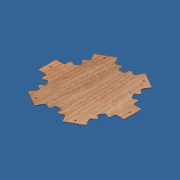
# Autodesk Inventor part: BaseTop
Saved by Autodesk Inventor 2014 SP2 (Build 180246200, 246)
## iProperties
Created: 2015-02-08
Part Number: BaseTop
Material: Holz (Birke)
Document SubType Name: Modeling
Designer: 4ndreas
Density: 0.55 g/cm^3
Appearance: Birke - natur - poliert
Author: 4ndreas
Autodesk Inventor part; units mm, degrees
ref_plane "YZ Plane" through (0, 0, 0) normal (1, 0, 0) x (0, 1, 0)
ref_plane "XZ Plane" through (0, 0, 0) normal (0, 1, 0) x (-1, 0, 0)
ref_plane "XY Plane" through (0, 0, 0) normal (0, 0, 1) x (1, 0, 0)
sketch "Skizze1" plane through (0, 0, 0) normal (0, 0, 1) x (1, 0, 0)
  arc A0 (67.0189, -1.4199) -> (65.1888, 5.4103) centre (62.6888, 1.0801) ccw projected
  line L0 (65.1888, 5.4103) -> (49.6003, 14.4103) projected
  line L1 (49.6003, 14.4103) -> (37.2798, 17.75) projected
  line L2 (37.2798, 17.75) -> (17.2798, 17.75) projected
  line L3 (17.2798, 17.75) -> (4.9593, 14.4103) projected
  line L4 (4.9593, 14.4103) -> (-10.6292, 5.4103) projected
  arc A1 (-10.6292, 5.4103) -> (-12.4593, -1.4199) centre (-8.1292, 1.0801) ccw projected
  line L5 (-12.4593, -1.4199) -> (-4.4593, -15.2763) projected
  arc A2 (-4.4593, -15.2763) -> (2.3708, -17.1064) centre (-0.1292, -12.7763) ccw projected
  line L6 (2.3708, -17.1064) -> (9.7798, -12.8288) projected
  arc A3 (17.2798, -17.159) -> (9.7798, -12.8288) centre (12.2798, -17.159) ccw projected
  line L7 (17.2798, -17.159) -> (17.2798, -23.4987) projected
  arc A4 (17.2798, -23.4987) -> (22.2798, -28.4987) centre (22.2798, -23.4987) ccw projected
  line L8 (22.2798, -28.4987) -> (32.2798, -28.4987) projected
  arc A5 (32.2798, -28.4987) -> (37.2798, -23.4987) centre (32.2798, -23.4987) ccw projected
  line L9 (37.2798, -23.4987) -> (37.2798, -17.159) projected
  arc A6 (44.7798, -12.8288) -> (37.2798, -17.159) centre (42.2798, -17.159) ccw projected
  line L10 (44.7798, -12.8288) -> (52.1888, -17.1064) projected
  arc A7 (52.1888, -17.1064) -> (59.0189, -15.2763) centre (54.6888, -12.7763) ccw projected
  line L11 (59.0189, -15.2763) -> (67.0189, -1.4199) projected
  circle A8 centre (27.2798, 7.75) radius 5.5 projected
  circle A9 centre (27.2798, -18.4987) radius 5.5 projected
  circle A10 centre (54.5596, 0) radius 5.5 projected
  circle A11 centre (0, 0) radius 5.5 projected
  arc A12 (-59.2247, -28.4199) -> (-66.0548, -26.5897) centre (-63.5548, -30.9199) ccw projected
  line L12 (-66.0548, -26.5897) -> (-81.6432, -35.5897) projected
  line L13 (-81.6432, -35.5897) -> (-90.6958, -44.5897) projected
  line L14 (-90.6958, -44.5897) -> (-100.6958, -61.9103) projected
  line L15 (-100.6958, -61.9103) -> (-103.9638, -74.25) projected
  line L16 (-103.9638, -74.25) -> (-103.9638, -92.25) projected
  arc A13 (-103.9638, -92.25) -> (-98.9638, -97.25) centre (-98.9638, -92.25) ccw projected
  line L17 (-98.9638, -97.25) -> (-82.9638, -97.25) projected
  arc A14 (-82.9638, -97.25) -> (-77.9638, -92.25) centre (-82.9638, -92.25) ccw projected
  line L18 (-77.9638, -92.25) -> (-77.9638, -83.6949) projected
  arc A15 (-70.4638, -79.3647) -> (-77.9638, -83.6949) centre (-72.9638, -83.6949) ccw projected
  line L19 (-70.4638, -79.3647) -> (-64.9734, -82.5346) projected
  arc A16 (-64.9734, -82.5346) -> (-58.1432, -80.7045) centre (-62.4734, -78.2045) ccw projected
  line L20 (-58.1432, -80.7045) -> (-53.1432, -72.0442) projected
  arc A17 (-53.1432, -72.0442) -> (-54.9734, -65.2141) centre (-57.4734, -69.5442) ccw projected
  line L21 (-54.9734, -65.2141) -> (-60.4638, -62.0442) projected
  arc A18 (-60.4638, -53.384) -> (-60.4638, -62.0442) centre (-57.9638, -57.7141) ccw projected
  line L22 (-60.4638, -53.384) -> (-53.0548, -49.1064) projected
  arc A19 (-53.0548, -49.1064) -> (-51.2247, -42.2763) centre (-55.5548, -44.7763) ccw projected
  line L23 (-51.2247, -42.2763) -> (-59.2247, -28.4199) projected
  circle A20 centre (-87.0356, -58.25) radius 5.5 projected
  circle A21 centre (-64.3035, -71.3744) radius 5.5 projected
  circle A22 centre (-66.684, -38.5) radius 5.5 projected
  circle A23 centre (-93.9638, -85.75) radius 5.5 projected
  arc A24 (-98.9638, -151.25) -> (-103.9638, -156.25) centre (-98.9638, -156.25) ccw projected
  line L24 (-103.9638, -156.25) -> (-103.9638, -174.25) projected
  line L25 (-103.9638, -174.25) -> (-100.6958, -186.5897) projected
  line L26 (-100.6958, -186.5897) -> (-90.6958, -203.9103) projected
  line L27 (-90.6958, -203.9103) -> (-81.6432, -212.9103) projected
  line L28 (-81.6432, -212.9103) -> (-66.0548, -221.9103) projected
  arc A25 (-66.0548, -221.9103) -> (-59.2247, -220.0801) centre (-63.5548, -217.5801) ccw projected
  line L29 (-59.2247, -220.0801) -> (-51.2247, -206.2237) projected
  arc A26 (-51.2247, -206.2237) -> (-53.0548, -199.3936) centre (-55.5548, -203.7237) ccw projected
  line L30 (-53.0548, -199.3936) -> (-60.4638, -195.116) projected
  arc A27 (-60.4638, -186.4558) -> (-60.4638, -195.116) centre (-57.9638, -190.7859) ccw projected
  line L31 (-60.4638, -186.4558) -> (-54.9734, -183.2859) projected
  arc A28 (-54.9734, -183.2859) -> (-53.1432, -176.4558) centre (-57.4734, -178.9558) ccw projected
  line L32 (-53.1432, -176.4558) -> (-58.1432, -167.7955) projected
  arc A29 (-58.1432, -167.7955) -> (-64.9734, -165.9654) centre (-62.4734, -170.2955) ccw projected
  line L33 (-64.9734, -165.9654) -> (-70.4638, -169.1353) projected
  arc A30 (-77.9638, -164.8051) -> (-70.4638, -169.1353) centre (-72.9638, -164.8051) ccw projected
  line L34 (-77.9638, -164.8051) -> (-77.9638, -156.25) projected
  arc A31 (-77.9638, -156.25) -> (-82.9638, -151.25) centre (-82.9638, -156.25) ccw projected
  line L35 (-82.9638, -151.25) -> (-98.9638, -151.25) projected
  circle A32 centre (-87.0356, -190.25) radius 5.5 projected
  circle A33 centre (-64.3035, -177.1256) radius 5.5 projected
  circle A34 centre (-93.9638, -162.75) radius 5.5 projected
  circle A35 centre (-66.684, -210) radius 5.5 projected
  arc A36 (-12.4593, -247.0801) -> (-10.6292, -253.9103) centre (-8.1292, -249.5801) ccw projected
  line L36 (-10.6292, -253.9103) -> (4.9593, -262.9103) projected
  line L37 (4.9593, -262.9103) -> (17.2798, -266.25) projected
  line L38 (17.2798, -266.25) -> (37.2798, -266.25) projected
  line L39 (37.2798, -266.25) -> (49.6003, -262.9103) projected
  line L40 (49.6003, -262.9103) -> (65.1888, -253.9103) projected
  arc A37 (65.1888, -253.9103) -> (67.0189, -247.0801) centre (62.6888, -249.5801) ccw projected
  line L41 (67.0189, -247.0801) -> (59.0189, -233.2237) projected
  arc A38 (59.0189, -233.2237) -> (52.1888, -231.3936) centre (54.6888, -235.7237) ccw projected
  line L42 (52.1888, -231.3936) -> (44.7798, -235.6712) projected
  arc A39 (37.2798, -231.341) -> (44.7798, -235.6712) centre (42.2798, -231.341) ccw projected
  line L43 (37.2798, -231.341) -> (37.2798, -225.0013) projected
  arc A40 (37.2798, -225.0013) -> (32.2798, -220.0013) centre (32.2798, -225.0013) ccw projected
  line L44 (32.2798, -220.0013) -> (22.2798, -220.0013) projected
  arc A41 (22.2798, -220.0013) -> (17.2798, -225.0013) centre (22.2798, -225.0013) ccw projected
  line L45 (17.2798, -225.0013) -> (17.2798, -231.341) projected
  arc A42 (9.7798, -235.6712) -> (17.2798, -231.341) centre (12.2798, -231.341) ccw projected
  line L46 (9.7798, -235.6712) -> (2.3708, -231.3936) projected
  arc A43 (2.3708, -231.3936) -> (-4.4593, -233.2237) centre (-0.1292, -235.7237) ccw projected
  line L47 (-4.4593, -233.2237) -> (-12.4593, -247.0801) projected
  circle A44 centre (27.2798, -256.25) radius 5.5 projected
  circle A45 centre (27.2798, -230.0013) radius 5.5 projected
  circle A46 centre (0, -248.5) radius 5.5 projected
  circle A47 centre (54.5596, -248.5) radius 5.5 projected
  arc A48 (113.7843, -220.0801) -> (120.6144, -221.9103) centre (118.1144, -217.5801) ccw projected
  line L48 (120.6144, -221.9103) -> (136.2028, -212.9103) projected
  line L49 (136.2028, -212.9103) -> (145.2554, -203.9103) projected
  line L50 (145.2554, -203.9103) -> (155.2554, -186.5897) projected
  line L51 (155.2554, -186.5897) -> (158.5234, -174.25) projected
  line L52 (158.5234, -174.25) -> (158.5234, -156.25) projected
  arc A49 (158.5234, -156.25) -> (153.5234, -151.25) centre (153.5234, -156.25) ccw projected
  line L53 (153.5234, -151.25) -> (137.5234, -151.25) projected
  arc A50 (137.5234, -151.25) -> (132.5234, -156.25) centre (137.5234, -156.25) ccw projected
  line L54 (132.5234, -156.25) -> (132.5234, -164.8051) projected
  arc A51 (125.0234, -169.1353) -> (132.5234, -164.8051) centre (127.5234, -164.8051) ccw projected
  line L55 (125.0234, -169.1353) -> (119.533, -165.9654) projected
  arc A52 (119.533, -165.9654) -> (112.7028, -167.7955) centre (117.033, -170.2955) ccw projected
  line L56 (112.7028, -167.7955) -> (107.7028, -176.4558) projected
  arc A53 (107.7028, -176.4558) -> (109.533, -183.2859) centre (112.033, -178.9558) ccw projected
  line L57 (109.533, -183.2859) -> (115.0234, -186.4558) projected
  arc A54 (115.0234, -195.116) -> (115.0234, -186.4558) centre (112.5234, -190.7859) ccw projected
  line L58 (115.0234, -195.116) -> (107.6144, -199.3936) projected
  arc A55 (107.6144, -199.3936) -> (105.7843, -206.2237) centre (110.1144, -203.7237) ccw projected
  line L59 (105.7843, -206.2237) -> (113.7843, -220.0801) projected
  circle A56 centre (141.5952, -190.25) radius 5.5 projected
  circle A57 centre (118.8631, -177.1256) radius 5.5 projected
  circle A58 centre (121.2436, -210) radius 5.5 projected
  circle A59 centre (148.5234, -162.75) radius 5.5 projected
  arc A60 (153.5234, -97.25) -> (158.5234, -92.25) centre (153.5234, -92.25) ccw projected
  line L60 (158.5234, -92.25) -> (158.5234, -74.25) projected
  line L61 (158.5234, -74.25) -> (155.2554, -61.9103) projected
  line L62 (155.2554, -61.9103) -> (145.2554, -44.5897) projected
  line L63 (145.2554, -44.5897) -> (136.2028, -35.5897) projected
  line L64 (136.2028, -35.5897) -> (120.6144, -26.5897) projected
  arc A61 (120.6144, -26.5897) -> (113.7843, -28.4199) centre (118.1144, -30.9199) ccw projected
  line L65 (113.7843, -28.4199) -> (105.7843, -42.2763) projected
  arc A62 (105.7843, -42.2763) -> (107.6144, -49.1064) centre (110.1144, -44.7763) ccw projected
  line L66 (107.6144, -49.1064) -> (115.0234, -53.384) projected
  arc A63 (115.0234, -62.0442) -> (115.0234, -53.384) centre (112.5234, -57.7141) ccw projected
  line L67 (115.0234, -62.0442) -> (109.533, -65.2141) projected
  arc A64 (109.533, -65.2141) -> (107.7028, -72.0442) centre (112.033, -69.5442) ccw projected
  line L68 (107.7028, -72.0442) -> (112.7028, -80.7045) projected
  arc A65 (112.7028, -80.7045) -> (119.533, -82.5346) centre (117.033, -78.2045) ccw projected
  line L69 (119.533, -82.5346) -> (125.0234, -79.3647) projected
  arc A66 (132.5234, -83.6949) -> (125.0234, -79.3647) centre (127.5234, -83.6949) ccw projected
  line L70 (132.5234, -83.6949) -> (132.5234, -92.25) projected
  arc A67 (132.5234, -92.25) -> (137.5234, -97.25) centre (137.5234, -92.25) ccw projected
  line L71 (137.5234, -97.25) -> (153.5234, -97.25) projected
  circle A68 centre (141.5952, -58.25) radius 5.5 projected
  circle A69 centre (118.8631, -71.3744) radius 5.5 projected
  circle A70 centre (148.5234, -85.75) radius 5.5 projected
  circle A71 centre (121.2436, -38.5) radius 5.5 projected
  line L72 (-37.254, -137.2494) -> (-38.7651, -138.1242) projected
  arc A72 (-38.7651, -138.1242) -> (-40.345, -144.0482) centre (-13.7095, -147.9791) ccw projected
  line L73 (-40.345, -144.0482) -> (-23.5645, -173.0347) projected
  arc A73 (-23.5645, -173.0347) -> (-17.6405, -174.6146) centre (-13.7095, -147.9791) ccw projected
  line L74 (-17.6405, -174.6146) -> (-16.1294, -173.7398) projected
  arc A74 (-16.1294, -173.7398) -> (-37.254, -137.2494) centre (27.2798, -124.25) ccw projected
  circle A75 centre (27.2798, -124.25) radius 80 projected
  arc A76 (-5.9641, -110.8301) -> (-4.134, -117.6603) centre (-1.634, -113.3301) ccw projected
  line L75 (-0.9641, -102.1699) -> (-5.9641, -110.8301) projected
  arc A77 (5.866, -100.3397) -> (-0.9641, -102.1699) centre (3.366, -104.6699) ccw projected
  line L76 (18.8564, -107.8397) -> (5.866, -100.3397) projected
  line L77 (35.7032, -107.8397) -> (18.8564, -107.8397) projected
  line L78 (35.7032, -107.8397) -> (48.6936, -100.3397) projected
  arc A78 (55.5237, -102.1699) -> (48.6936, -100.3397) centre (51.1936, -104.6699) ccw projected
  line L79 (60.5237, -110.8301) -> (55.5237, -102.1699) projected
  arc A79 (58.6936, -117.6603) -> (60.5237, -110.8301) centre (56.1936, -113.3301) ccw projected
  line L80 (45.7032, -125.1603) -> (58.6936, -117.6603) projected
  line L81 (37.2798, -139.75) -> (45.7032, -125.1603) projected
  line L82 (37.2798, -139.75) -> (37.2798, -154.75) projected
  arc A80 (32.2798, -159.75) -> (37.2798, -154.75) centre (32.2798, -154.75) ccw projected
  line L83 (22.2798, -159.75) -> (32.2798, -159.75) projected
  arc A81 (17.2798, -154.75) -> (22.2798, -159.75) centre (22.2798, -154.75) ccw projected
  line L84 (17.2798, -139.75) -> (17.2798, -154.75) projected
  line L85 (8.8564, -125.1603) -> (17.2798, -139.75) projected
  line L86 (8.8564, -125.1603) -> (-4.134, -117.6603) projected
  circle A82 centre (27.2798, -149.75) radius 5.5 projected
  circle A83 centre (49.3634, -111.5) radius 5.5 projected
  circle A84 centre (5.1962, -111.5) radius 5.5 projected
  circle A85 centre (27.2798, -124.25) radius 11.5 projected
  arc A86 (-38.7651, -138.1242) -> (-40.345, -144.0482) centre (-13.7095, -147.9791) ccw projected
  line L87 (-9.7786, -121.3436) -> (-38.7651, -138.1242) projected
  arc A87 (-3.8546, -122.9235) -> (-9.7786, -121.3436) centre (-13.7095, -147.9791) ccw projected
  line L88 (12.926, -151.91) -> (-3.8546, -122.9235) projected
  arc A88 (11.346, -157.8341) -> (12.926, -151.91) centre (-13.7095, -147.9791) ccw projected
  line L89 (-17.6405, -174.6146) -> (11.346, -157.8341) projected
  arc A89 (-23.5645, -173.0347) -> (-17.6405, -174.6146) centre (-13.7095, -147.9791) ccw projected
  line L90 (-40.345, -144.0482) -> (-23.5645, -173.0347) projected
  arc A90 (-15.9365, -144.1322) -> (-11.4825, -151.826) centre (-13.7095, -147.9791) ccw projected
  arc A91 (-11.4825, -151.826) -> (-15.9365, -144.1322) centre (-13.7095, -147.9791) ccw projected
  line L91 (137.5234, -150.65) -> (153.5234, -150.65)
  arc A92 (159.1234, -156.25) -> (153.5234, -150.65) centre (153.5234, -156.25) ccw
  line L92 (159.1234, -156.25) -> (159.1234, -174.3281)
  line L93 (159.1234, -174.3281) -> (155.815, -186.8206)
  line L94 (155.815, -186.8206) -> (145.7351, -204.2794)
  line L95 (145.7351, -204.2794) -> (136.5705, -213.3908)
  line L96 (136.5705, -213.3908) -> (120.9144, -222.4299)
  arc A93 (113.2646, -220.3801) -> (120.9144, -222.4299) centre (118.1144, -217.5801) ccw
  line L97 (113.2646, -220.3801) -> (105.2646, -206.5237)
  arc A94 (107.3144, -198.874) -> (105.2646, -206.5237) centre (110.1144, -203.7237) ccw
  line L98 (107.3144, -198.874) -> (114.7234, -194.5964)
  arc A95 (114.7234, -194.5964) -> (114.7234, -186.9754) centre (112.5234, -190.7859) ccw
  line L99 (114.7234, -186.9754) -> (109.233, -183.8055)
  arc A96 (107.1832, -176.1558) -> (109.233, -183.8055) centre (112.033, -178.9558) ccw
  line L100 (107.1832, -176.1558) -> (112.1832, -167.4955)
  arc A97 (119.833, -165.4458) -> (112.1832, -167.4955) centre (117.033, -170.2955) ccw
  line L101 (119.833, -165.4458) -> (125.3234, -168.6156)
  arc A98 (125.3234, -168.6156) -> (131.9234, -164.8051) centre (127.5234, -164.8051) ccw
  line L102 (131.9234, -164.8051) -> (131.9234, -156.25)
  arc A99 (137.5234, -150.65) -> (131.9234, -156.25) centre (137.5234, -156.25) ccw
  line L103 (131.9234, -92.25) -> (131.9234, -83.6949)
  arc A100 (131.9234, -83.6949) -> (125.3234, -79.8844) centre (127.5234, -83.6949) ccw
  line L104 (125.3234, -79.8844) -> (119.833, -83.0542)
  arc A101 (112.1832, -81.0045) -> (119.833, -83.0542) centre (117.033, -78.2045) ccw
  line L105 (112.1832, -81.0045) -> (107.1832, -72.3442)
  arc A102 (109.233, -64.6945) -> (107.1832, -72.3442) centre (112.033, -69.5442) ccw
  line L106 (109.233, -64.6945) -> (114.7234, -61.5246)
  arc A103 (114.7234, -61.5246) -> (114.7234, -53.9036) centre (112.5234, -57.7141) ccw
  line L107 (114.7234, -53.9036) -> (107.3144, -49.626)
  arc A104 (105.2646, -41.9763) -> (107.3144, -49.626) centre (110.1144, -44.7763) ccw
  line L108 (105.2646, -41.9763) -> (113.2646, -28.1199)
  arc A105 (120.9144, -26.0701) -> (113.2646, -28.1199) centre (118.1144, -30.9199) ccw
  line L109 (120.9144, -26.0701) -> (136.5705, -35.1092)
  line L110 (136.5705, -35.1092) -> (145.7351, -44.2206)
  line L111 (145.7351, -44.2206) -> (155.815, -61.6794)
  line L112 (155.815, -61.6794) -> (159.1234, -74.1719)
  line L113 (159.1234, -74.1719) -> (159.1234, -92.25)
  arc A106 (153.5234, -97.85) -> (159.1234, -92.25) centre (153.5234, -92.25) ccw
  line L114 (153.5234, -97.85) -> (137.5234, -97.85)
  arc A107 (131.9234, -92.25) -> (137.5234, -97.85) centre (137.5234, -92.25) ccw
  line L115 (16.6798, -23.4987) -> (16.6798, -17.159)
  arc A108 (16.6798, -17.159) -> (10.0798, -13.3485) centre (12.2798, -17.159) ccw
  line L116 (10.0798, -13.3485) -> (2.6708, -17.626)
  arc A109 (-4.9789, -15.5763) -> (2.6708, -17.626) centre (-0.1292, -12.7763) ccw
  line L117 (-4.9789, -15.5763) -> (-12.9789, -1.7199)
  arc A110 (-10.9292, 5.9299) -> (-12.9789, -1.7199) centre (-8.1292, 1.0801) ccw
  line L118 (-10.9292, 5.9299) -> (4.7269, 14.9689)
  line L119 (4.7269, 14.9689) -> (17.1999, 18.35)
  line L120 (17.1999, 18.35) -> (37.3597, 18.35)
  line L121 (37.3597, 18.35) -> (49.8327, 14.9689)
  line L122 (49.8327, 14.9689) -> (65.4888, 5.9299)
  arc A111 (67.5385, -1.7199) -> (65.4888, 5.9299) centre (62.6888, 1.0801) ccw
  line L123 (67.5385, -1.7199) -> (59.5385, -15.5763)
  arc A112 (51.8888, -17.626) -> (59.5385, -15.5763) centre (54.6888, -12.7763) ccw
  line L124 (51.8888, -17.626) -> (44.4798, -13.3485)
  arc A113 (44.4798, -13.3485) -> (37.8798, -17.159) centre (42.2798, -17.159) ccw
  line L125 (37.8798, -17.159) -> (37.8798, -23.4987)
  arc A114 (32.2798, -29.0987) -> (37.8798, -23.4987) centre (32.2798, -23.4987) ccw
  line L126 (32.2798, -29.0987) -> (22.2798, -29.0987)
  arc A115 (16.6798, -23.4987) -> (22.2798, -29.0987) centre (22.2798, -23.4987) ccw
  arc A116 (-52.7548, -49.626) -> (-50.705, -41.9763) centre (-55.5548, -44.7763) ccw
  line L127 (-52.7548, -49.626) -> (-60.1638, -53.9036)
  arc A117 (-60.1638, -53.9036) -> (-60.1638, -61.5246) centre (-57.9638, -57.7141) ccw
  line L128 (-60.1638, -61.5246) -> (-54.6734, -64.6945)
  arc A118 (-52.6236, -72.3442) -> (-54.6734, -64.6945) centre (-57.4734, -69.5442) ccw
  line L129 (-52.6236, -72.3442) -> (-57.6236, -81.0045)
  arc A119 (-65.2734, -83.0542) -> (-57.6236, -81.0045) centre (-62.4734, -78.2045) ccw
  line L130 (-65.2734, -83.0542) -> (-70.7638, -79.8844)
  arc A120 (-70.7638, -79.8844) -> (-77.3638, -83.6949) centre (-72.9638, -83.6949) ccw
  line L131 (-77.3638, -83.6949) -> (-77.3638, -92.25)
  arc A121 (-82.9638, -97.85) -> (-77.3638, -92.25) centre (-82.9638, -92.25) ccw
  line L132 (-82.9638, -97.85) -> (-98.9638, -97.85)
  arc A122 (-104.5638, -92.25) -> (-98.9638, -97.85) centre (-98.9638, -92.25) ccw
  line L133 (-104.5638, -92.25) -> (-104.5638, -74.1719)
  line L134 (-104.5638, -74.1719) -> (-101.2554, -61.6794)
  line L135 (-101.2554, -61.6794) -> (-91.1755, -44.2206)
  line L136 (-91.1755, -44.2206) -> (-82.0109, -35.1092)
  line L137 (-82.0109, -35.1092) -> (-66.3548, -26.0701)
  arc A123 (-58.705, -28.1199) -> (-66.3548, -26.0701) centre (-63.5548, -30.9199) ccw
  line L138 (-58.705, -28.1199) -> (-50.705, -41.9763)
  arc A124 (59.5385, -232.9237) -> (51.8888, -230.874) centre (54.6888, -235.7237) ccw
  line L139 (59.5385, -232.9237) -> (67.5385, -246.7801)
  arc A125 (65.4888, -254.4299) -> (67.5385, -246.7801) centre (62.6888, -249.5801) ccw
  line L140 (65.4888, -254.4299) -> (49.8327, -263.4689)
  line L141 (49.8327, -263.4689) -> (37.3597, -266.85)
  line L142 (37.3597, -266.85) -> (17.1999, -266.85)
  line L143 (17.1999, -266.85) -> (4.7269, -263.4689)
  line L144 (4.7269, -263.4689) -> (-10.9292, -254.4299)
  arc A126 (-12.9789, -246.7801) -> (-10.9292, -254.4299) centre (-8.1292, -249.5801) ccw
  line L145 (-12.9789, -246.7801) -> (-4.9789, -232.9237)
  arc A127 (2.6708, -230.874) -> (-4.9789, -232.9237) centre (-0.1292, -235.7237) ccw
  line L146 (2.6708, -230.874) -> (10.0798, -235.1515)
  arc A128 (10.0798, -235.1515) -> (16.6798, -231.341) centre (12.2798, -231.341) ccw
  line L147 (16.6798, -231.341) -> (16.6798, -225.0013)
  arc A129 (22.2798, -219.4013) -> (16.6798, -225.0013) centre (22.2798, -225.0013) ccw
  line L148 (22.2798, -219.4013) -> (32.2798, -219.4013)
  arc A130 (37.8798, -225.0013) -> (32.2798, -219.4013) centre (32.2798, -225.0013) ccw
  line L149 (37.8798, -225.0013) -> (37.8798, -231.341)
  arc A131 (37.8798, -231.341) -> (44.4798, -235.1515) centre (42.2798, -231.341) ccw
  line L150 (44.4798, -235.1515) -> (51.8888, -230.874)
  line L151 (-66.3548, -222.4299) -> (-82.0109, -213.3908)
  line L152 (-82.0109, -213.3908) -> (-91.1755, -204.2794)
  line L153 (-91.1755, -204.2794) -> (-101.2554, -186.8206)
  line L154 (-101.2554, -186.8206) -> (-104.5638, -174.3281)
  line L155 (-104.5638, -174.3281) -> (-104.5638, -156.25)
  arc A132 (-98.9638, -150.65) -> (-104.5638, -156.25) centre (-98.9638, -156.25) ccw
  line L156 (-98.9638, -150.65) -> (-82.9638, -150.65)
  arc A133 (-77.3638, -156.25) -> (-82.9638, -150.65) centre (-82.9638, -156.25) ccw
  line L157 (-77.3638, -156.25) -> (-77.3638, -164.8051)
  arc A134 (-77.3638, -164.8051) -> (-70.7638, -168.6156) centre (-72.9638, -164.8051) ccw
  line L158 (-70.7638, -168.6156) -> (-65.2734, -165.4458)
  arc A135 (-57.6236, -167.4955) -> (-65.2734, -165.4458) centre (-62.4734, -170.2955) ccw
  line L159 (-57.6236, -167.4955) -> (-52.6236, -176.1558)
  arc A136 (-54.6734, -183.8055) -> (-52.6236, -176.1558) centre (-57.4734, -178.9558) ccw
  line L160 (-54.6734, -183.8055) -> (-60.1638, -186.9754)
  arc A137 (-60.1638, -186.9754) -> (-60.1638, -194.5964) centre (-57.9638, -190.7859) ccw
  line L161 (-60.1638, -194.5964) -> (-52.7548, -198.874)
  arc A138 (-50.705, -206.5237) -> (-52.7548, -198.874) centre (-55.5548, -203.7237) ccw
  line L162 (-50.705, -206.5237) -> (-58.705, -220.3801)
  arc A139 (-66.3548, -222.4299) -> (-58.705, -220.3801) centre (-63.5548, -217.5801) ccw
  line L163 (158.5234, -153.7281) -> (158.5234, -94.7719)
  line L164 (118.4304, -25.3288) -> (67.3728, 4.1493)
  line L165 (-12.8132, 4.1493) -> (-63.8708, -25.3288)
  line L166 (-103.9638, -153.7281) -> (-103.9638, -94.7719)
  line L167 (-12.8132, -252.6493) -> (-63.8708, -223.1712)
  line L168 (118.4304, -223.1712) -> (67.3728, -252.6493)
  point P0 (0, 0)
  dimension "d0" = 0.6
  dimension "d1" = 0.6
  dimension "d2" = 0.6
  dimension "d3" = 0.6
  dimension "d4" = 0.6
  dimension "d5" = 0.6
  constraints: 156 end point, 108 point on circle, 48 centre point, 7 collinear, 2 parallel, 114 other
  measures "d0" distance between parallel lines of L53 L91
  measures "d1" distance between parallel lines of L41 L139
  measures "d2" distance between parallel lines of L162 L29
  measures "d3" distance between parallel lines of L132 L17
  measures "d4" distance between parallel lines of L117 L5
  measures "d5" distance between parallel lines of L114 L71
extrude "Extrusion1" add sketch "Skizze1" against normal blind 3 contours A75 | A99 L102 A98 L101 A97 L100 A96 L99 A95 L98 A94 L97 A93 L168 A125 L139 A124 L150 A131 L149 A130 L148 A129 L147 A128 L146 A127 L145 A126 L167 A139 L162 A138 L161 A137 L160 A136 L159 A135 L158 A134 L157 A133 L156 A132 L166 A122 L132 A121 L131 A120 L130 A119 L129 A118 L128 A117 L127 A116 L138 A123 L165 A110 L117 A109 L116 A108 L115 A115 L126 A114 L125 A113 L124 A112 L123 A111 L164 A105 L108 A104 L107 A103 L106 A102 L105 A101 L104 A100 L103 A107 L114 A106 L163 A92 L91
fillet "Rundung1" radius 2 12 edges at (158.5234, -153.7281, -1.5) (158.5234, -94.7719, -1.5) (118.4304, -25.3288, -1.5) (67.3728, 4.1493, -1.5) (-12.8132, 4.1493, -1.5) (-63.8708, -25.3288, -1.5) (-103.9638, -94.7719, -1.5) (-103.9638, -153.7281, -1.5) (-63.8708, -223.1712, -1.5) (-12.8132, -252.6493, -1.5) (67.3728, -252.6493, -1.5) (118.4304, -223.1712, -1.5)
sketch "Skizze2" plane through (0, 0, 0) normal (0, 0, 1) x (1, 0, 0)
  arc A0 (-38.7651, -138.1242) -> (-40.345, -144.0482) centre (-13.7095, -147.9791) ccw
  line L0 (-38.7651, -138.1242) -> (-37.254, -137.2494)
  arc A1 (-16.1294, -173.7398) -> (-37.254, -137.2494) centre (27.2798, -124.25) ccw
  line L1 (-16.1294, -173.7398) -> (-17.6405, -174.6146)
  arc A2 (-23.5645, -173.0347) -> (-17.6405, -174.6146) centre (-13.7095, -147.9791) ccw
  line L2 (-23.5645, -173.0347) -> (-40.345, -144.0482)
  circle A3 centre (27.2798, -124.25) radius 80
  circle A4 centre (27.1946, -51.335) radius 3.3
  circle A5 centre (90.3834, -87.7187) radius 3.3
  circle A6 centre (90.4686, -160.6337) radius 3.3
  circle A7 centre (27.365, -197.165) radius 3.3
  circle A8 centre (-35.8238, -160.7813) radius 3.3
  circle A9 centre (-35.909, -87.8663) radius 3.3
  arc A10 (50.9479, -139.702) -> (49.0131, -139.363) centre (49.4912, -142.3246) ccw
  line L3 (49.0131, -139.363) -> (40.732, -140.7)
  arc A11 (19.7134, -104.3927) -> (40.732, -140.7) centre (27.2798, -124.25) ccw
  line L4 (19.7134, -104.3927) -> (24.9966, -97.8772)
  arc A12 (24.9966, -97.8772) -> (25.666, -96.0305) centre (22.6663, -95.9877) ccw
  line L5 (25.666, -96.0305) -> (26.1574, -61.5981)
  arc A13 (26.1574, -61.5981) -> (22.9609, -58.5618) centre (23.1577, -61.5553) ccw
  arc A14 (22.9609, -58.5618) -> (-37.7935, -134.203) centre (27.2798, -124.25) ccw
  arc A15 (-39.256, -137.2529) -> (-37.7935, -134.203) centre (-40.759, -134.6566) ccw
  line L6 (-39.256, -137.2529) -> (-39.565, -137.4317)
  arc A16 (-39.565, -137.4317) -> (-41.3835, -144.2504) centre (-13.7095, -147.9791) ccw
  line L7 (-41.3835, -144.2504) -> (-24.2569, -173.8345)
  arc A17 (-24.2569, -173.8345) -> (-17.4383, -175.6531) centre (-13.7095, -147.9791) ccw
  line L8 (-17.4383, -175.6531) -> (-17.1293, -175.4742)
  arc A18 (-13.7562, -175.7247) -> (-17.1293, -175.4742) centre (-15.6263, -178.0705) ccw
  arc A19 (-13.7562, -175.7247) -> (82.0934, -160.7064) centre (27.2798, -124.25) ccw
  arc A20 (82.0934, -160.7064) -> (81.0521, -156.4224) centre (79.5954, -159.045) ccw
  line L9 (81.0521, -156.4224) -> (50.9479, -139.702)
  arc A21 (27.6684, -95.8821) -> (28.3749, -97.8591) centre (30.6681, -95.9249) ccw
  line L10 (28.3749, -97.8591) -> (32.9449, -103.2773)
  arc A22 (32.9449, -103.2773) -> (34.2535, -104.1769) centre (35.2381, -101.343) ccw
  arc A23 (48.1598, -128.1983) -> (34.2535, -104.1769) centre (27.2798, -124.25) ccw
  arc A24 (48.1598, -128.1983) -> (48.2882, -129.7812) centre (51.1075, -128.7557) ccw
  line L11 (48.2882, -129.7812) -> (50.7111, -136.4424)
  arc A25 (50.7111, -136.4424) -> (52.0737, -138.0395) centre (53.5304, -135.4169) ccw
  line L12 (52.0737, -138.0395) -> (82.1365, -154.7369)
  arc A26 (82.1365, -154.7369) -> (86.282, -153.4447) centre (83.5932, -152.1143) ccw
  arc A27 (86.282, -153.4447) -> (31.344, -58.5455) centre (27.2798, -124.25) ccw
  arc A28 (31.344, -58.5455) -> (28.1591, -61.497) centre (31.1587, -61.5398) ccw
  line L13 (28.1591, -61.497) -> (27.6684, -95.8821)
  circle A29 centre (-35.8238, -160.7813) radius 3.3
  circle A30 centre (90.4686, -160.6337) radius 3.3
  circle A31 centre (27.1946, -51.335) radius 3.3
  circle A32 centre (90.3834, -87.7187) radius 3.3
  circle A33 centre (27.365, -197.165) radius 3.3
  circle A34 centre (-35.909, -87.8663) radius 3.3
  circle A35 centre (27.2798, -124.25) radius 80
  circle A36 centre (27.2798, -124.25) radius 11.25
  point P0 (0, 0)
extrude "Extrusion2" cut sketch "Skizze2" against normal through all contours L0 A1 A13 L5 A12 L4 A11 L3 A10 L9 A20 L1 A2 L2 A0 | A0 L2 A2 L1 A1 A18 L8 A17 L7 A16 L6 A15 L0 | A4 | A5 | A6 | A7 | A8 | A9
sketch "Skizze3" plane through (0, 0, 0) normal (0, 0, 1) x (1, 0, 0)
  line L0 (158.5234, -149.2672) -> (158.5234, -99.2328) projected
  line L1 (-103.9638, -99.2328) -> (-103.9638, -149.2672) projected
  line L2 (158.5234, -124.25) -> (-103.9638, -124.25) construction
  point P0 (0, 0)
  point P1 (148.5234, -124.25)
  dimension "d11" = 10
  constraints: 2 end point, 2 midpoint, 1 point on line
  measures "d11" distance from line of L0 point (148.523, -124.25)
hole "Bohrung1" at (148.5234, -124.25, 0) direction (0, 0, -1) diameter 5 depth 8 tip angle 118
pattern_circular "Runde Anordnung1" count 6 over 360 about axis through (27.2798, -124.25, 0) along (0, 0, -1) of "Bohrung1"
sketch "Skizze4" plane through (0, 0, 0) normal (0, 0, 1) x (1, 0, 0)
  arc A0 (-13.7562, -175.7247) -> (-17.1293, -175.4742) centre (-15.6263, -178.0705) ccw projected
  line L0 (-17.1293, -175.4742) -> (-17.4383, -175.6531) projected
  arc A1 (-24.2569, -173.8345) -> (-17.4383, -175.6531) centre (-13.7095, -147.9791) ccw projected
  line L1 (-24.2569, -173.8345) -> (-41.3835, -144.2504) projected
  arc A2 (-39.565, -137.4317) -> (-41.3835, -144.2504) centre (-13.7095, -147.9791) ccw projected
  line L2 (-39.565, -137.4317) -> (-39.256, -137.2529) projected
  arc A3 (-39.256, -137.2529) -> (-37.7935, -134.203) centre (-40.759, -134.6566) ccw projected
  arc A4 (-13.7562, -175.7247) -> (-37.7935, -134.203) centre (27.2798, -124.25) ccw projected
  circle A5 centre (-35.909, -87.8663) radius 3.3 projected
  circle A6 centre (27.365, -197.165) radius 3.3 projected
  circle A7 centre (90.3834, -87.7187) radius 3.3 projected
  circle A8 centre (27.1946, -51.335) radius 3.3 projected
  circle A9 centre (90.4686, -160.6337) radius 3.3 projected
  circle A10 centre (-35.8238, -160.7813) radius 3.3 projected
  point P0 (0, 0)
extrude "Extrusion3" add sketch "Skizze4" against normal up to surface (3 mm away)
equation "\"d1\" = d0"
equation "\"d2\" = d1"
equation "\"d3\" = d2"
equation "\"d4\" = d3"
equation "\"d5\" = d0"
